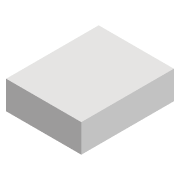
# Autodesk Inventor part: Part79
Saved by Autodesk Inventor 2020.5 (Build 245400000, 400)
## iProperties
Created: 2022-11-26
Part Number: Part79
Material: 一般
Document SubType Name: Modeling
Designer: Administrator
Density: 1 g/cm^3
Appearance: 既定
Author: Administrator
Autodesk Inventor part; units mm, degrees
ref_plane "YZ Plane" through (0, 0, 0) normal (1, 0, 0) x (0, 1, 0)
ref_plane "XZ Plane" through (0, 0, 0) normal (0, 1, 0) x (-1, 0, 0)
ref_plane "XY Plane" through (0, 0, 0) normal (0, 0, 1) x (1, 0, 0)
sketch "スケッチ1" plane through (0, 0, 0) normal (0, 0, 1) x (1, 0, 0)
  line L0 (-39.0005, 72.869) -> (120.9986, 72.869) projected
  line L1 (120.9986, 72.869) -> (120.9986, -75.131) projected
  line L2 (120.9986, -75.131) -> (-39.0005, -75.131) projected
  line L3 (-39.0005, -75.131) -> (-39.0005, 72.869) projected
  circle A0 centre (-24.0923, 43.869) radius 6 projected
  circle A1 centre (106.0905, 43.869) radius 6 projected
  circle A2 centre (-24.0923, 28.369) radius 3 projected
  circle A3 centre (-24.0923, 59.369) radius 3 projected
  circle A4 centre (106.0905, 28.369) radius 3 projected
  circle A5 centre (106.0905, 59.369) radius 3 projected
  line L4 (120.9986, -75.131) -> (120.9986, -15.131)
  line L5 (120.9986, -15.131) -> (-39.0014, -15.131)
  line L6 (-39.0014, -15.131) -> (-39.0014, -75.131)
  line L7 (-39.0014, -75.131) -> (120.9986, -75.131)
  point P0 (0, 0)
  point P1 (-39.0005, -15.131)
  dimension "d0" = 60
  dimension "d1" = 160
  constraints: 8 end point, 2 parallel, 1 perpendicular, 1 point on line
  measures "d0" distance of L1.end L4.end
  measures "d1" distance of L5.end L4.end
extrude "押し出し1" add sketch "スケッチ1" along normal blind 197 contours L5 L1 L2 L3
sketch "スケッチ2" plane through (-39.0005, -75.131, 0) normal (0, -1, 0) x (1, 0, 0)
  line L0 (0, 0) -> (159.9991, 0) projected
  line L1 (159.9991, 0) -> (159.9991, 197) projected
  line L2 (0, 197) -> (159.9991, 197) projected
  line L3 (0, 0) -> (0, 197) projected
  line L4 (139.9991, 182) -> (139.9991, 15)
  line L5 (139.9991, 15) -> (20, 15)
  line L6 (20, 15) -> (20, 182)
  line L7 (20, 182) -> (139.9991, 182)
  line L8 (159.9991, 0) -> (159.9991, 197) projected
  line L9 (0, 0) -> (0, 197) projected
  line L10 (0, 197) -> (159.9991, 197) projected
  line L11 (0, 0) -> (159.9991, 0) projected
  point P0 (39.0005, 0)
  dimension "d4" = 20
  dimension "d5" = 20
  dimension "d6" = 15
  dimension "d7" = 15
  constraints: 8 end point, 2 parallel, 1 perpendicular, 1 vertical
  measures "d4" distance between parallel lines of L4 L8
  measures "d5" distance between parallel lines of L6 L9
  measures "d6" distance between parallel lines of L7 L10
  measures "d7" distance between parallel lines of L11 L5
